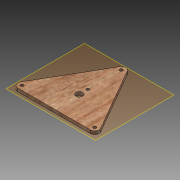
# Autodesk Inventor part: ServoHousingEndPlates
Saved by Autodesk Inventor 2014 SP1 (Build 180222100, 222)
## iProperties
Created: 2014-11-03
Part Number: ServoHousingEndPlates
Material: Wood (Birch)
Document SubType Name: Modeling
Designer: rawrdong
Density: 0.55 g/cm^3
Appearance: Birch - Natural Polished
Author: rawrdong
Autodesk Inventor part; units mm, degrees
ref_plane "YZ Plane" through (0, 0, 0) normal (1, 0, 0) x (0, 1, 0)
ref_plane "XZ Plane" through (0, 0, 0) normal (0, 1, 0) x (-1, 0, 0)
ref_plane "XY Plane" through (0, 0, 0) normal (0, 0, 1) x (1, 0, 0)
ref_plane "Work Plane1" through (0, 0, 0) normal (0, 0, 1) x (1, 0, 0)
sketch "Sketch1" plane through (0, 0, 0) normal (0, 0, 1) x (1, 0, 0)
  circle A0 centre (-34, 58.3124) radius 1.425 projected
  circle A1 centre (-67.5, 0.2887) radius 1.425 projected
  circle A2 centre (-0.5, 0.2887) radius 1.425 projected
  arc A3 (-2.5, 3.7528) -> (-4.5, 0.2887) centre (-0.5, 0.2887) ccw projected
  arc A4 (-5, -0.2113) -> (-4.5, 0.2887) centre (-5, 0.2887) ccw projected
  line L0 (-5, -0.2113) -> (-63, -0.2113) projected
  arc A5 (-63.5, 0.2887) -> (-63, -0.2113) centre (-63, 0.2887) ccw projected
  arc A6 (-63.5, 0.2887) -> (-65.5, 3.7528) centre (-67.5, 0.2887) ccw projected
  arc A7 (-65.683, 4.4358) -> (-65.5, 3.7528) centre (-65.25, 4.1858) ccw projected
  line L1 (-65.683, 4.4358) -> (-36.683, 54.6653) projected
  arc A8 (-36, 54.8483) -> (-36.683, 54.6653) centre (-36.25, 54.4153) ccw projected
  arc A9 (-36, 54.8483) -> (-32, 54.8483) centre (-34, 58.3124) ccw projected
  arc A10 (-31.317, 54.6653) -> (-32, 54.8483) centre (-31.75, 54.4153) ccw projected
  line L2 (-31.317, 54.6653) -> (-2.317, 4.4358) projected
  arc A11 (-2.5, 3.7528) -> (-2.317, 4.4358) centre (-2.75, 4.1858) ccw projected
  line L3 (2.9641, 2.2887) -> (-30.5359, 60.3124) projected
  arc A12 (-30.5359, 60.3124) -> (-37.4641, 60.3124) centre (-34, 58.3124) ccw projected
  line L4 (-37.4641, 60.3124) -> (-70.9641, 2.2887) projected
  arc A13 (-70.9641, 2.2887) -> (-67.5, -3.7113) centre (-67.5, 0.2887) ccw projected
  line L5 (-67.5, -3.7113) -> (-0.5, -3.7113) projected
  arc A14 (-0.5, -3.7113) -> (2.9641, 2.2887) centre (-0.5, 0.2887) ccw projected
  circle A15 centre (-34, 58.3124) radius 1.45
  circle A16 centre (-0.5, 0.2887) radius 1.45
  circle A17 centre (-67.5, 0.2887) radius 1.45
  line L6 (-67.5, 0.2887) -> (-13.7859, 31.3005) construction
  line L7 (-0.5, 0.2887) -> (-54.2141, 31.3005) construction
  point P0 (0, 0)
  point P1 (-34, 19.6299)
  dimension "d0" = 2.9
  constraints: 4 end point, 3 centre point, 3 coincident, 2 equal radius, 2 midpoint, 2 point on line
  measures "d0" diameter of A15
extrude "Extrusion1" add sketch "Sketch1" along normal blind 3 contours A3 A4 L0 A5 A6 A7 L1 A8 A9 A10 L2 A11 | A14 L5 A13 L4 A12 L3
sketch "Sketch2" plane through (0, 0, 3) normal (0, 0, 1) x (1, 0, 0)
  line L0 (2.9641, 2.2887) -> (-30.5359, 60.3124) projected
  arc A0 (-30.5359, 60.3124) -> (-37.4641, 60.3124) centre (-34, 58.3124) ccw projected
  line L1 (-34, 58.3124) -> (-34, -3.7946) construction
  circle A1 centre (-34, 19.6299) radius 3.175
  circle A2 centre (-67.5, 0.2887) radius 1.45 projected
  line L2 (-67.5, 0.2887) -> (-13.7859, 31.3005) construction
  circle A3 centre (-34, 27.5299) radius 1.425
  dimension "d33" = 6.35
  dimension "d34" = 2.85
  dimension "d35" = 7.9
  constraints: 4 end point, 4 point on line, 2 centre point, 1 coincident, 1 midpoint, 1 vertical
  measures "d33" diameter of A1
  measures "d34" diameter of A3
  measures "d35" distance of A1.centre A3.centre
extrude "Extrusion4" cut sketch "Sketch2" against normal through all contours A1 | A3
body "Solid1"
